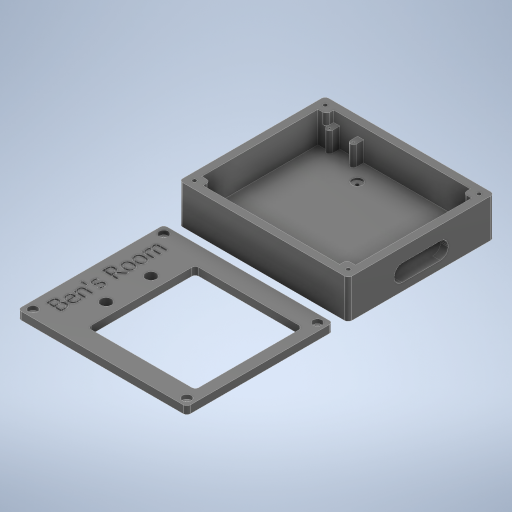
# Autodesk Inventor part: Front Circuit Box
Saved by Autodesk Inventor 2024 (Build 280153000, 153)
## iProperties
Created: 2024-01-30
Part Number: Front Circuit Box
Material: ABS Plastic
Document SubType Name: Modeling
Designer: himmelb
Density: 1.06 g/cm^3
Appearance: Smooth - Black
Author: himmelb
Autodesk Inventor part; units mm, degrees
ref_plane "YZ Plane" through (0, 0, 0) normal (1, 0, 0) x (0, 1, 0)
ref_plane "XZ Plane" through (0, 0, 0) normal (0, 1, 0) x (-1, 0, 0)
ref_plane "XY Plane" through (0, 0, 0) normal (0, 0, 1) x (1, 0, 0)
sketch "Sketch1" plane through (0, 0, 0) normal (0, 1, 0) x (-1, 0, 0)
  line L0 (0, 0) -> (110, 0)
  line L1 (110, 0) -> (110, -95)
  line L2 (110, -95) -> (0, -95)
  line L3 (0, -95) -> (0, 0)
  dimension "d0" = 110
  dimension "d1" = 95
  constraints: 8 end point, 2 parallel, 1 horizontal, 1 perpendicular
  measures "d0" distance of L1.end L2.end
  measures "d1" distance of L0.end L1.end
extrude "Extrusion1" add sketch "Sketch1" along normal blind 25
shell "Shell1" thickness 5 removed faces 1 at (-36.6667, 25, -31.6667)
sketch "Sketch2" plane through (-105, 5, -90) normal (0, 1, 0) x (1, 0, 0)
  circle A0 centre (92, -72.1) radius 3.5
  circle A1 centre (92, -12.9) radius 3.5
  circle A2 centre (33.73, -72.0689) radius 3.5
  circle A3 centre (33.73, -12.9) radius 3.5
  line L0 (100, -85) -> (0, -85) projected
  line L1 (0, 0) -> (100, 0) projected
  line L2 (100, 0) -> (100, -85) projected
  point P0 (105, -90)
  dimension "d8" = 58.27
  dimension "d9" = 12.9
  dimension "d10" = 12.9
  dimension "d11" = 8
  dimension "d13" = 8
  dimension "d15" = 7
  dimension "d16" = 7
  dimension "d17" = 7
  dimension "d18" = 7
  constraints: 4 centre point
  measures "d8" distance of A0.centre A2.centre
  measures "d9" distance from line of A0.centre L0
  measures "d10" distance from line of L1 A1.centre
  measures "d11" distance from line of L2 A0.centre
  measures "d13" distance from line of L2 A1.centre
  measures "d15" diameter of A2
  measures "d16" diameter of A3
  measures "d17" diameter of A0
  measures "d18" diameter of A1
extrude "Extrusion2" cut sketch "Sketch2" against normal blind 1.5
sketch "Sketch3" plane through (0, 0, 0) normal (0, -1, 0) x (1, 0, 0)
  circle A0 centre (-13, -17.9) radius 3.5 projected
  circle A1 centre (-13, -17.9) radius 3.5
  circle A2 centre (-13, -77.1) radius 3.5 projected
  circle A3 centre (-13, -77.1) radius 3.5
  circle A4 centre (-71.27, -77.1) radius 3.5 projected
  circle A5 centre (-71.27, -77.1) radius 3.5
  circle A6 centre (-71.27, -17.9311) radius 3.5 projected
  circle A7 centre (-71.27, -17.9311) radius 3.5
  point P0 (0, 0)
  constraints: 4 centre point, 4 coincident
extrude "Extrusion3" cut sketch "Sketch3" against normal blind 1.5
sketch "Sketch4" plane through (-71.27, 3.5, -77.1) normal (0, 1, 0) x (1, 0, 0)
  circle A0 centre (0, 0) radius 3.5 projected
  circle A1 centre (0, 0) radius 1.25
  circle A2 centre (0, -59.1689) radius 3.5 projected
  circle A3 centre (0, -59.1689) radius 1.25
  circle A4 centre (58.27, -59.2) radius 3.5 projected
  circle A5 centre (58.27, -59.2) radius 1.25
  circle A6 centre (58.27, 0) radius 3.5 projected
  circle A7 centre (58.27, 0) radius 1.25
  point P0 (71.27, -77.1)
  dimension "d24" = 2.5
  dimension "d25" = 2.5
  dimension "d26" = 2.5
  dimension "d27" = 2.5
  constraints: 4 centre point, 4 coincident
  measures "d24" diameter of A1
  measures "d25" diameter of A7
  measures "d26" diameter of A5
  measures "d27" diameter of A3
extrude "Extrusion4" cut sketch "Sketch4" against normal blind 2 contours A1 | A3 | A5 | A7
sketch "Sketch5" plane through (0, 0, 0) normal (1, 0, 0) x (0, 0, -1)
  line L0 (95, 0) -> (0, 0) projected
  line L1 (65, 5) -> (65, 16.0603)
  line L2 (65, 16.0603) -> (30, 16.0603)
  line L3 (30, 16.0603) -> (30, 5)
  line L4 (0, 0) -> (0, 25) projected
  line L5 (30, 5) -> (65, 5)
  dimension "d33" = 35
  dimension "d34" = 30
  dimension "d35" = 5
  constraints: 8 end point, 1 parallel, 1 perpendicular
  measures "d33" distance between parallel lines of L1 L3
  measures "d34" distance between parallel lines of L4 L3
  measures "d35" distance between parallel lines of L5 L0
extrude "Extrusion5" cut sketch "Sketch5" against normal blind 5
sketch "Sketch6" plane through (-105, 5, -90) normal (0, 1, 0) x (1, 0, 0)
  circle A0 centre (33.73, -72.0689) radius 3.5 projected
  line L0 (0, 0) -> (0, -85) projected
  circle A1 centre (33.73, -12.9) radius 3.5 projected
  line L1 (100, -85) -> (0, -85) projected
  line L2 (0, 0) -> (100, 0) projected
  arc A2 (9.5575, -80.25) -> (5.5575, -80.25) centre (7.5575, -80.25) ccw
  arc A3 (25.0575, -80.25) -> (21.0575, -80.25) centre (23.0575, -80.25) ccw
  arc A4 (21.0575, -4.75) -> (25.0575, -4.75) centre (23.0575, -4.75) ccw
  arc A5 (5.5575, -4.75) -> (9.5575, -4.75) centre (7.5575, -4.75) ccw
  line L3 (25.0575, -80.25) -> (25.0575, -85)
  line L4 (25.0575, -85) -> (5.5575, -85)
  line L5 (5.5575, -85) -> (5.5575, -80.25)
  line L6 (25.0575, -4.75) -> (25.0575, 0)
  line L7 (25.0575, 0) -> (5.5575, 0)
  line L8 (5.5575, 0) -> (5.5575, -4.75)
  line L9 (9.5575, -80.25) -> (9.5575, -85)
  line L10 (21.0575, -80.25) -> (21.0575, -85)
  line L11 (21.0575, -4.75) -> (21.0575, 0)
  line L12 (9.5575, -4.75) -> (9.5575, 0)
  line L13 (5.5575, -80.25) -> (9.5575, -80.25)
  line L14 (21.0575, -80.25) -> (25.0575, -80.25)
  point P0 (105, -90)
  point P1 (21.0575, -85)
  point P2 (5.5575, -85)
  point P3 (9.5575, -85)
  point P4 (21.0575, 0)
  dimension "d39" = 4.75
  dimension "d40" = 4.75
  dimension "d41" = 4.75
  dimension "d42" = 4.75
  dimension "d43" = 15.5
  dimension "d44" = 15.5
  dimension "d45" = 4
  dimension "d46" = 4
  dimension "d47" = 4
  dimension "d48" = 4
  constraints: 24 end point, 9 point on line, 8 point on circle, 4 centre point, 4 coincident, 4 parallel, 3 perpendicular, 2 horizontal, 2 tangent
  measures "d39" distance from line of L1 point (7.558, -80.25)
  measures "d40" distance from line of L2 point (7.558, -4.75)
  measures "d41" distance from line of L2 point (23.058, -4.75)
  measures "d42" distance from line of L1 point (23.058, -80.25)
  measures "d43" distance of point (23.058, -80.25) point (7.558, -80.25)
  measures "d44" distance of point (23.058, -4.75) point (7.558, -4.75)
  measures "d45" diameter of A5
  measures "d46" diameter of A4
  measures "d47" diameter of A3
  measures "d48" diameter of A2
extrude "Extrusion6" add sketch "Sketch6" along normal blind 13 contours L1 L10 L14 L3 | L14 A3 | L1 L5 L13 L9 | L13 A2 | L2 L12 A5 L8 | L2 L6 A4 L11
sketch "Sketch7" plane through (-97.4425, 18, -9.75) normal (0, 1, 0) x (-1, 0, 0)
  circle A0 centre (0, 0) radius 0.64
  arc A1 (-17.5, 0) -> (-13.5, 0) centre (-15.5, 0) ccw projected
  circle A2 centre (-15.5, 0) radius 0.64
  arc A3 (2, -75.5) -> (-2, -75.5) centre (0, -75.5) ccw projected
  circle A4 centre (0, -75.5) radius 0.64
  arc A5 (-13.5, -75.5) -> (-17.5, -75.5) centre (-15.5, -75.5) ccw projected
  circle A6 centre (-15.5, -75.5) radius 0.64
  point P0 (-97.4425, 9.75)
  point P1 (15.5, 0)
  point P2 (15.5, 75.5)
  point P3 (0, 75.5)
  dimension "d51" = 1.28
  dimension "d52" = 1.28
  dimension "d53" = 1.28
  dimension "d54" = 1.28
  constraints: 4 centre point, 4 coincident
  measures "d51" diameter of A6
  measures "d52" diameter of A4
  measures "d53" diameter of A2
  measures "d54" diameter of A0
extrude "Extrusion7" cut sketch "Sketch7" against normal blind 5.4
sketch "Sketch8" plane through (0, 25, 0) normal (0, 1, 0) x (1, 0, 0)
  line L0 (-105, 5) -> (-105, 90) projected
  arc A0 (-95.4425, 9.75) -> (-99.4425, 9.75) centre (-97.4425, 9.75) ccw projected
  line L1 (-105, 5) -> (-99.4425, 5)
  line L2 (-99.4425, 5) -> (-99.4425, 9.75)
  line L3 (-99.4425, 9.75) -> (-105, 9.75)
  line L4 (-105, 9.75) -> (-105, 5)
  arc A1 (-99.4425, 85.25) -> (-95.4425, 85.25) centre (-97.4425, 85.25) ccw projected
  line L5 (-105, 90) -> (-99.4425, 90)
  line L6 (-99.4425, 90) -> (-99.4425, 85.25)
  line L7 (-99.4425, 85.25) -> (-105, 85.25)
  line L8 (-105, 85.25) -> (-105, 90)
  line L9 (-105, 5) -> (-5, 5) projected
  line L10 (-55, 5) -> (-55, 90)
  line L11 (-5, 90) -> (-105, 90) projected
  line L12 (-5, 5) -> (-10.5575, 5)
  line L13 (-10.5575, 5) -> (-10.5575, 9.75)
  line L14 (-10.5575, 9.75) -> (-5, 9.75)
  line L15 (-5, 9.75) -> (-5, 5)
  line L16 (-5, 90) -> (-10.5575, 90)
  line L17 (-10.5575, 90) -> (-10.5575, 85.25)
  line L18 (-10.5575, 85.25) -> (-5, 85.25)
  line L19 (-5, 85.25) -> (-5, 90)
  line L20 (-5, 5) -> (-5, 9.75)
  line L21 (-5, 85.25) -> (-5, 90)
  point P0 (0, 0)
  constraints: 38 end point, 6 symmetric about line, 4 parallel, 2 horizontal, 2 midpoint, 2 perpendicular, 2 point on circle
extrude "Extrusion8" add sketch "Sketch8" against normal blind 20 contours L0 L3 L2 L1 | L0 L5 L6 L7 | L13 L14 L15 L9 | L19 L18 L17 L11
fillet "Fillet1" radius 5.08 4 edges at (-2.5, 16.0603, -65) (-2.5, 16.0603, -30) (-2.5, 5, -30) (-2.5, 5, -65)
sketch "Sketch9" plane through (0, 25, 0) normal (0, 1, 0) x (1, 0, 0)
  circle A0 centre (-105, 90) radius 1.335
  circle A1 centre (-5, 90) radius 1.335
  circle A2 centre (-5, 5) radius 1.335
  circle A3 centre (-105, 5) radius 1.335
  line L0 (-99.4425, 85.25) -> (-99.4425, 90) projected
  line L1 (-105, 85.25) -> (-99.4425, 85.25) projected
  point P0 (0, 0)
  point P1 (-102.2212, 85.25)
  dimension "d65" = 2.67
  dimension "d66" = 2.67
  dimension "d67" = 2.67
  dimension "d68" = 2.67
  constraints: 4 centre point, 1 midpoint
  measures "d65" diameter of A0
  measures "d66" diameter of A1
  measures "d67" diameter of A2
  measures "d68" diameter of A3
extrude "Extrusion9" cut sketch "Sketch9" against normal blind 20
sketch "Sketch10" plane through (0, 0, 0) normal (0, -1, 0) x (1, 0, 0)
  line L0 (0, 105) -> (-110, 105)
  line L1 (-110, 105) -> (-110, 10)
  line L2 (-110, 10) -> (0, 10)
  line L3 (0, 10) -> (0, 105)
  line L4 (0, 0) -> (0, -95) projected
  line L5 (-110, 0) -> (0, 0) projected
  dimension "d71" = 95
  dimension "d72" = 110
  dimension "d73" = 0
  dimension "d74" = 10
  constraints: 8 end point, 2 parallel, 1 horizontal, 1 perpendicular
  measures "d71" distance between parallel lines of L2 L0
  measures "d72" distance of L1.end L2.end
  measures "d73" distance between parallel lines of L3 L4
  measures "d74" distance between parallel lines of L5 L2
extrude "Extrusion10" add sketch "Sketch10" against normal blind 5
sketch "Sketch11" plane through (0, 5, 0) normal (0, 1, 0) x (1, 0, 0)
  circle A0 centre (-105, -15) radius 1.335
  circle A1 centre (-5, -15) radius 1.335
  circle A2 centre (-5, -100) radius 1.335
  circle A3 centre (-105, -100) radius 1.335
  line L0 (0, -10) -> (-110, -10) projected
  line L1 (0, -105) -> (0, -10) projected
  line L2 (-110, -105) -> (0, -105) projected
  line L3 (-110, -10) -> (-110, -105) projected
  circle A4 centre (-105, -15) radius 3
  circle A5 centre (-5, -15) radius 3
  circle A6 centre (-5, -100) radius 3
  circle A7 centre (-105, -100) radius 3
  point P0 (0, 0)
  dimension "d77" = 5
  dimension "d78" = 5
  dimension "d79" = 5
  dimension "d80" = 5
  dimension "d81" = 5
  dimension "d82" = 5
  dimension "d83" = 5
  dimension "d84" = 5
  dimension "d85" = 2.67
  dimension "d86" = 2.67
  dimension "d87" = 2.67
  dimension "d88" = 2.67
  dimension "d89" = 6
  dimension "d90" = 6
  dimension "d91" = 6
  dimension "d92" = 6
  constraints: 8 centre point, 4 coincident
  measures "d77" distance from line of L0 A1.centre
  measures "d78" distance from line of L1 A1.centre
  measures "d79" distance from line of L2 A2.centre
  measures "d80" distance from line of L1 A2.centre
  measures "d81" distance from line of L2 A3.centre
  measures "d82" distance from line of L3 A3.centre
  measures "d83" distance from line of L3 A0.centre
  measures "d84" distance from line of L0 A0.centre
  measures "d85" diameter of A3
  measures "d86" diameter of A0
  measures "d87" diameter of A1
  measures "d88" diameter of A2
  measures "d89" diameter of A4
  measures "d90" diameter of A5
  measures "d91" diameter of A6
  measures "d92" diameter of A7
extrude "Extrusion11" cut sketch "Sketch11" against normal blind 2.7 contours A0 | A1 | A2 | A3 | A4 | A5 | A6 | A7
sketch "Sketch12" plane through (0, 5, 0) normal (0, 1, 0) x (1, 0, 0)
  circle A0 centre (-105, -100) radius 3 projected
  circle A1 centre (-105, -100) radius 1.335
  circle A2 centre (-105, -15) radius 3 projected
  circle A3 centre (-105, -15) radius 1.335
  circle A4 centre (-5, -15) radius 3 projected
  circle A5 centre (-5, -15) radius 1.335
  circle A6 centre (-5, -100) radius 3 projected
  circle A7 centre (-5, -100) radius 1.335
  line L0 (-110, -10) -> (-110, -105) projected
  point P0 (0, 0)
  dimension "d95" = 2.67
  dimension "d96" = 2.67
  dimension "d97" = 2.67
  dimension "d98" = 2.67
  constraints: 4 centre point, 4 coincident
  measures "d95" diameter of A1
  measures "d96" diameter of A3
  measures "d97" diameter of A5
  measures "d98" diameter of A7
extrude "Extrusion12" cut sketch "Sketch12" against normal blind 5 contours A1 | A3 | A5 | A7
sketch "Sketch13" plane through (0, 5, 0) normal (0, 1, 0) x (1, 0, 0)
  line L0 (-77, -22.5) -> (-7, -22.5)
  line L1 (-7, -22.5) -> (-7, -92.5)
  line L2 (-7, -92.5) -> (-77, -92.5)
  line L3 (-77, -92.5) -> (-77, -22.5)
  line L4 (0, -10) -> (-110, -10) projected
  line L5 (0, -105) -> (0, -10) projected
  circle A0 centre (-13, 17.9) radius 3.5 projected
  circle A1 centre (-71.27, 17.9311) radius 3.5 projected
  circle A2 centre (-85.4425, -42.89) radius 3.5
  circle A3 centre (-85.4425, -72.11) radius 3.5
  line L6 (-110, -105) -> (0, -105) projected
  circle A4 centre (-81.9425, 9.75) radius 0.64 projected
  circle A5 centre (-97.4425, 9.75) radius 0.64 projected
  point P0 (0, 0)
  dimension "d101" = 70
  dimension "d102" = 70
  dimension "d103" = 12.5
  dimension "d104" = 7
  dimension "d105" = 7
  dimension "d106" = 7
  dimension "d107" = 32.89
  dimension "d108" = 32.89
  dimension "d110" = 3.5
  dimension "d111" = 3.5
  constraints: 8 end point, 3 coincident, 2 centre point, 2 parallel, 1 horizontal, 1 perpendicular
  measures "d101" distance between parallel lines of L2 L0
  measures "d102" distance of L0.start L0.end
  measures "d103" distance between parallel lines of L4 L0
  measures "d104" distance between parallel lines of L5 L1
  measures "d105" diameter of A2
  measures "d106" diameter of A3
  measures "d107" distance from line of L4 A2.centre
  measures "d108" distance from line of L6 A3.centre
  measures "d110" horizontal distance of A2.centre point (-81.942, 9.75)
  measures "d111" horizontal distance of point (-81.942, 9.75) A3.centre
extrude "Extrusion13" cut sketch "Sketch13" against normal blind 5 contours L0 L1 L2 L3 | A2 | A3
fillet "Fillet3" radius 2.25 16 edges at (0, 2.5, 105) (0, 2.5, 10) (-110, 2.5, 105) (-77, 2.5, 22.5) (-7, 2.5, 22.5) (-7, 2.5, 92.5) (-77, 2.5, 92.5) (-110, 2.5, 10) (-110, 12.5, -95) (0, 12.5, -95) (-110, 12.5, 0) (0, 12.5, 0) (-99.4425, 21.5, -9.75) (-99.4425, 21.5, -85.25) (-10.5575, 15, -85.25) (-10.5575, 15, -9.75)
sketch "Sketch14" plane through (0, 5, 0) normal (0, 1, 0) x (1, 0, 0)
  line L0 (-105, -95) -> (-105, -20) construction
  line L1 (-105, -20) -> (-90.6726, -20) construction
  line L2 (-90.6726, -20) -> (-90.6726, -95) construction
  line L3 (-90.6726, -95) -> (-105, -95) construction
  line L4 (-110, -12.25) -> (-110, -102.75) projected
  line L5 (-107.75, -105) -> (-2.25, -105) projected
  line L6 (-2.25, -10) -> (-107.75, -10) projected
  spline S0 degree 2 poles (-97.62, -85.398) (-96.8739, -85.398) (-95.7304, -85.9657) (-95.3573, -86.4361) knots 0 0 0 1 2 2 2
  spline S1 degree 2 poles (-95.3573, -86.4361) (-94.9194, -87.0038) (-94.5464, -88.2932) (-94.5464, -89.3151) knots 0 0 0 1 2 2 2
  line L7 (-94.5464, -89.3151) -> (-94.5464, -92.186)
  line L8 (-94.5464, -92.186) -> (-104.554, -92.186)
  line L9 (-104.554, -92.186) -> (-104.554, -89.534)
  spline S2 degree 2 poles (-104.554, -89.534) (-104.554, -88.4635) (-104.4161, -87.393) (-104.1485, -86.9064) knots 0 0 0 1 2 2 2
  spline S3 degree 2 poles (-104.1485, -86.9064) (-103.8646, -86.3631) (-102.932, -85.8684) (-102.2994, -85.8684) knots 0 0 0 1 2 2 2
  spline S4 degree 2 poles (-102.2994, -85.8684) (-101.5938, -85.8684) (-100.4747, -86.6145) (-100.1584, -87.2714) knots 0 0 0 1 2 2 2
  line L10 (-100.1584, -87.2714) -> (-100.1097, -87.2714)
  spline S5 degree 2 poles (-100.1097, -87.2714) (-99.8664, -86.3793) (-98.577, -85.398) (-97.62, -85.398) knots 0 0 0 1 2 2 2
  spline S6 degree 2 poles (-97.5632, -86.7848) (-98.1309, -86.7848) (-98.8608, -87.1092) (-99.1203, -87.5958) knots 0 0 0 1 2 2 2
  spline S7 degree 2 poles (-99.1203, -87.5958) (-99.2825, -87.9121) (-99.3798, -88.6582) (-99.3798, -89.3475) knots 0 0 0 1 2 2 2
  line L11 (-99.3798, -89.3475) -> (-99.3798, -90.856)
  line L12 (-99.3798, -90.856) -> (-95.6817, -90.856)
  line L13 (-95.6817, -90.856) -> (-95.6817, -89.7773)
  spline S8 degree 2 poles (-95.6817, -89.7773) (-95.6817, -88.9015) (-95.8439, -87.8959) (-96.1035, -87.5066) knots 0 0 0 1 2 2 2
  spline S9 degree 2 poles (-96.1035, -87.5066) (-96.3711, -87.1335) (-97.0361, -86.7848) (-97.5632, -86.7848) knots 0 0 0 1 2 2 2
  spline S10 degree 2 poles (-102.1129, -87.2552) (-102.4697, -87.2552) (-103.005, -87.4985) (-103.1591, -87.7661) knots 0 0 0 1 2 2 2
  spline S11 degree 2 poles (-103.1591, -87.7661) (-103.3375, -88.0905) (-103.4186, -88.8771) (-103.4186, -89.5827) knots 0 0 0 1 2 2 2
  line L14 (-103.4186, -89.5827) -> (-103.4186, -90.856)
  line L15 (-103.4186, -90.856) -> (-100.4909, -90.856)
  line L16 (-100.4909, -90.856) -> (-100.4909, -89.3475)
  spline S12 degree 2 poles (-100.4909, -89.3475) (-100.4909, -88.7231) (-100.6207, -88.131) (-100.8234, -87.8148) knots 0 0 0 1 2 2 2
  spline S13 degree 2 poles (-100.8234, -87.8148) (-101.018, -87.5066) (-101.6425, -87.2552) (-102.1129, -87.2552) knots 0 0 0 1 2 2 2
  spline S14 degree 2 poles (-94.376, -80.9132) (-94.376, -82.7136) (-96.3954, -84.6924) (-98.2607, -84.6924) knots 0 0 0 1 2 2 2
  spline S15 degree 2 poles (-98.2607, -84.6924) (-100.0935, -84.6924) (-102.267, -82.7704) (-102.267, -81.2214) knots 0 0 0 1 2 2 2
  spline S16 degree 2 poles (-102.267, -81.2214) (-102.267, -80.524) (-101.8615, -79.4454) (-101.4317, -79.048) knots 0 0 0 1 2 2 2
  spline S17 degree 2 poles (-101.4317, -79.048) (-101.0018, -78.6425) (-99.761, -78.2126) (-98.8608, -78.2126) knots 0 0 0 1 2 2 2
  line L17 (-98.8608, -78.2126) -> (-98.1715, -78.2126)
  line L18 (-98.1715, -78.2126) -> (-98.1715, -83.4111)
  spline S18 degree 2 poles (-98.1715, -83.4111) (-96.8658, -83.4111) (-95.479, -82.0973) (-95.479, -80.9295) knots 0 0 0 1 2 2 2
  spline S19 degree 2 poles (-95.479, -80.9295) (-95.479, -80.5159) (-95.6655, -79.713) (-95.8115, -79.3886) knots 0 0 0 1 2 2 2
  spline S20 degree 2 poles (-95.8115, -79.3886) (-95.9737, -79.048) (-96.2575, -78.5776) (-96.3873, -78.4235) knots 0 0 0 1 2 2 2
  line L19 (-96.3873, -78.4235) -> (-96.3873, -78.3505)
  line L20 (-96.3873, -78.3505) -> (-95.0086, -78.3505)
  spline S21 degree 2 poles (-95.0086, -78.3505) (-94.9194, -78.5695) (-94.6599, -79.2345) (-94.5869, -79.494) knots 0 0 0 1 2 2 2
  spline S22 degree 2 poles (-94.5869, -79.494) (-94.4815, -79.859) (-94.376, -80.4591) (-94.376, -80.9132) knots 0 0 0 1 2 2 2
  spline S23 degree 2 poles (-99.1366, -79.4454) (-99.6475, -79.4616) (-100.3936, -79.6724) (-100.645, -79.8752) knots 0 0 0 1 2 2 2
  spline S24 degree 2 poles (-100.645, -79.8752) (-100.9288, -80.0941) (-101.2289, -80.7835) (-101.2289, -81.2944) knots 0 0 0 1 2 2 2
  spline S25 degree 2 poles (-101.2289, -81.2944) (-101.2289, -81.7972) (-100.9288, -82.5028) (-100.6369, -82.7947) knots 0 0 0 1 2 2 2
  spline S26 degree 2 poles (-100.6369, -82.7947) (-100.3368, -83.0786) (-99.615, -83.3705) (-99.1366, -83.4111) knots 0 0 0 1 2 2 2
  line L21 (-99.1366, -83.4111) -> (-99.1366, -79.4454)
  line L22 (-94.5464, -71.0354) -> (-94.5464, -72.3005)
  line L23 (-94.5464, -72.3005) -> (-98.8284, -72.3005)
  spline S27 degree 2 poles (-98.8284, -72.3005) (-99.3474, -72.3005) (-100.2395, -72.3979) (-100.5071, -72.5438) knots 0 0 0 1 2 2 2
  spline S28 degree 2 poles (-100.5071, -72.5438) (-100.791, -72.6979) (-101.0667, -73.2494) (-101.0667, -73.7198) knots 0 0 0 1 2 2 2
  spline S29 degree 2 poles (-101.0667, -73.7198) (-101.0667, -74.1901) (-100.5639, -75.1877) (-100.1584, -75.6661) knots 0 0 0 1 2 2 2
  line L24 (-100.1584, -75.6661) -> (-94.5464, -75.6661)
  line L25 (-94.5464, -75.6661) -> (-94.5464, -76.9313)
  line L26 (-94.5464, -76.9313) -> (-102.0561, -76.9313)
  line L27 (-102.0561, -76.9313) -> (-102.0561, -75.6661)
  line L28 (-102.0561, -75.6661) -> (-101.2208, -75.6661)
  spline S30 degree 2 poles (-101.2208, -75.6661) (-101.7317, -75.0985) (-102.267, -74.0036) (-102.267, -73.3873) knots 0 0 0 1 2 2 2
  spline S31 degree 2 poles (-102.267, -73.3873) (-102.267, -72.2843) (-100.8072, -71.0354) (-99.4204, -71.0354) knots 0 0 0 1 2 2 2
  line L29 (-99.4204, -71.0354) -> (-94.5464, -71.0354)
  line L30 (-105, -67.978) -> (-101.1073, -68.2699)
  line L31 (-101.1073, -68.2699) -> (-101.1073, -69.1782)
  line L32 (-101.1073, -69.1782) -> (-105, -69.4702)
  line L33 (-105, -69.4702) -> (-105, -67.978)
  spline S32 degree 2 poles (-94.3679, -64.3285) (-94.3679, -65.0827) (-94.7734, -66.3884) (-95.0005, -66.8183) knots 0 0 0 1 2 2 2
  line L34 (-95.0005, -66.8183) -> (-96.4197, -66.8183)
  line L35 (-96.4197, -66.8183) -> (-96.4197, -66.7534)
  spline S33 degree 2 poles (-96.4197, -66.7534) (-96.29, -66.5912) (-95.9818, -66.1532) (-95.8115, -65.7883) knots 0 0 0 1 2 2 2
  spline S34 degree 2 poles (-95.8115, -65.7883) (-95.6574, -65.472) (-95.4303, -64.6935) (-95.4303, -64.2799) knots 0 0 0 1 2 2 2
  spline S35 degree 2 poles (-95.4303, -64.2799) (-95.4303, -63.9798) (-95.5682, -63.2905) (-95.6817, -63.1283) knots 0 0 0 1 2 2 2
  spline S36 degree 2 poles (-95.6817, -63.1283) (-95.8358, -62.8931) (-96.1846, -62.6822) (-96.5414, -62.6822) knots 0 0 0 1 2 2 2
  spline S37 degree 2 poles (-96.5414, -62.6822) (-96.9874, -62.6822) (-97.4497, -63.1688) (-97.6038, -63.7933) knots 0 0 0 1 2 2 2
  spline S38 degree 2 poles (-97.6038, -63.7933) (-97.6606, -64.0366) (-97.8228, -64.8151) (-97.912, -65.1476) knots 0 0 0 1 2 2 2
  spline S39 degree 2 poles (-97.912, -65.1476) (-98.1634, -66.0073) (-99.2014, -66.7858) (-99.9394, -66.7858) knots 0 0 0 1 2 2 2
  spline S40 degree 2 poles (-99.9394, -66.7858) (-100.9613, -66.7858) (-102.2345, -65.2531) (-102.2345, -63.9879) knots 0 0 0 1 2 2 2
  spline S41 degree 2 poles (-102.2345, -63.9879) (-102.2345, -63.3634) (-101.9264, -62.0983) (-101.6912, -61.6685) knots 0 0 0 1 2 2 2
  line L36 (-101.6912, -61.6685) -> (-100.3368, -61.6685)
  line L37 (-100.3368, -61.6685) -> (-100.3368, -61.7334)
  spline S42 degree 2 poles (-100.3368, -61.7334) (-100.7261, -62.22) (-101.1721, -63.404) (-101.1721, -64.0122) knots 0 0 0 1 2 2 2
  spline S43 degree 2 poles (-101.1721, -64.0122) (-101.1721, -64.6367) (-100.645, -65.4963) (-100.1178, -65.4963) knots 0 0 0 1 2 2 2
  spline S44 degree 2 poles (-100.1178, -65.4963) (-99.6394, -65.4963) (-99.1771, -64.9854) (-99.0311, -64.4177) knots 0 0 0 1 2 2 2
  spline S45 degree 2 poles (-99.0311, -64.4177) (-98.9581, -64.142) (-98.8122, -63.4445) (-98.7229, -63.0634) knots 0 0 0 1 2 2 2
  spline S46 degree 2 poles (-98.7229, -63.0634) (-98.5121, -62.2362) (-97.547, -61.3927) (-96.7117, -61.3927) knots 0 0 0 1 2 2 2
  spline S47 degree 2 poles (-96.7117, -61.3927) (-96.2251, -61.3927) (-95.3655, -61.7739) (-95.0492, -62.147) knots 0 0 0 1 2 2 2
  spline S48 degree 2 poles (-95.0492, -62.147) (-94.7167, -62.5443) (-94.3679, -63.5581) (-94.3679, -64.3285) knots 0 0 0 1 2 2 2
  line L38 (-94.5464, -48.0763) -> (-94.5464, -49.8037)
  line L39 (-94.5464, -49.8037) -> (-98.5283, -52.9666)
  line L40 (-98.5283, -52.9666) -> (-98.5283, -54.4912)
  line L41 (-98.5283, -54.4912) -> (-94.5464, -54.4912)
  line L42 (-94.5464, -54.4912) -> (-94.5464, -55.8213)
  line L43 (-94.5464, -55.8213) -> (-104.554, -55.8213)
  line L44 (-104.554, -55.8213) -> (-104.554, -53.2423)
  spline S49 degree 2 poles (-104.554, -53.2423) (-104.554, -52.3827) (-104.3674, -51.2229) (-104.0268, -50.6958) knots 0 0 0 1 2 2 2
  spline S50 degree 2 poles (-104.0268, -50.6958) (-103.6862, -50.1687) (-102.6238, -49.5604) (-101.8371, -49.5604) knots 0 0 0 1 2 2 2
  spline S51 degree 2 poles (-101.8371, -49.5604) (-100.7423, -49.5604) (-99.2582, -50.6796) (-98.9014, -51.6366) knots 0 0 0 1 2 2 2
  line L45 (-98.9014, -51.6366) -> (-94.5464, -48.0763)
  spline S52 degree 2 poles (-101.7317, -50.9472) (-102.1697, -50.9472) (-102.8428, -51.2554) (-103.0617, -51.5798) knots 0 0 0 1 2 2 2
  spline S53 degree 2 poles (-103.0617, -51.5798) (-103.2483, -51.8636) (-103.4024, -52.6178) (-103.4024, -53.1693) knots 0 0 0 1 2 2 2
  line L46 (-103.4024, -53.1693) -> (-103.4024, -54.4912)
  line L47 (-103.4024, -54.4912) -> (-99.6394, -54.4912)
  line L48 (-99.6394, -54.4912) -> (-99.6394, -53.3234)
  spline S54 degree 2 poles (-99.6394, -53.3234) (-99.6394, -52.7476) (-99.8421, -51.8312) (-100.1584, -51.5149) knots 0 0 0 1 2 2 2
  spline S55 degree 2 poles (-100.1584, -51.5149) (-100.4341, -51.2229) (-101.2127, -50.9472) (-101.7317, -50.9472) knots 0 0 0 1 2 2 2
  spline S56 degree 2 poles (-98.3012, -41.2072) (-96.4035, -41.2072) (-94.3355, -43.032) (-94.3355, -44.5566) knots 0 0 0 1 2 2 2
  spline S57 degree 2 poles (-94.3355, -44.5566) (-94.3355, -46.1218) (-96.4684, -47.9141) (-98.3012, -47.9141) knots 0 0 0 1 2 2 2
  spline S58 degree 2 poles (-98.3012, -47.9141) (-100.1827, -47.9141) (-102.267, -46.0651) (-102.267, -44.5566) knots 0 0 0 1 2 2 2
  spline S59 degree 2 poles (-102.267, -44.5566) (-102.267, -43.032) (-100.1908, -41.2072) (-98.3012, -41.2072) knots 0 0 0 1 2 2 2
  spline S60 degree 2 poles (-98.3012, -42.5129) (-99.761, -42.5129) (-101.1802, -43.5753) (-101.1802, -44.5566) knots 0 0 0 1 2 2 2
  spline S61 degree 2 poles (-101.1802, -44.5566) (-101.1802, -45.5379) (-99.761, -46.6084) (-98.3012, -46.6084) knots 0 0 0 1 2 2 2
  spline S62 degree 2 poles (-98.3012, -46.6084) (-96.882, -46.6084) (-95.4222, -45.5379) (-95.4222, -44.5566) knots 0 0 0 1 2 2 2
  spline S63 degree 2 poles (-95.4222, -44.5566) (-95.4222, -43.5834) (-96.8577, -42.5129) (-98.3012, -42.5129) knots 0 0 0 1 2 2 2
  spline S64 degree 2 poles (-98.3012, -33.738) (-96.4035, -33.738) (-94.3355, -35.5628) (-94.3355, -37.0874) knots 0 0 0 1 2 2 2
  spline S65 degree 2 poles (-94.3355, -37.0874) (-94.3355, -38.6526) (-96.4684, -40.4449) (-98.3012, -40.4449) knots 0 0 0 1 2 2 2
  spline S66 degree 2 poles (-98.3012, -40.4449) (-100.1827, -40.4449) (-102.267, -38.5959) (-102.267, -37.0874) knots 0 0 0 1 2 2 2
  spline S67 degree 2 poles (-102.267, -37.0874) (-102.267, -35.5628) (-100.1908, -33.738) (-98.3012, -33.738) knots 0 0 0 1 2 2 2
  spline S68 degree 2 poles (-98.3012, -35.0437) (-99.761, -35.0437) (-101.1802, -36.1061) (-101.1802, -37.0874) knots 0 0 0 1 2 2 2
  spline S69 degree 2 poles (-101.1802, -37.0874) (-101.1802, -38.0687) (-99.761, -39.1392) (-98.3012, -39.1392) knots 0 0 0 1 2 2 2
  spline S70 degree 2 poles (-98.3012, -39.1392) (-96.882, -39.1392) (-95.4222, -38.0687) (-95.4222, -37.0874) knots 0 0 0 1 2 2 2
  spline S71 degree 2 poles (-95.4222, -37.0874) (-95.4222, -36.1142) (-96.8577, -35.0437) (-98.3012, -35.0437) knots 0 0 0 1 2 2 2
  line L49 (-94.5464, -23.9251) -> (-98.8933, -23.9251)
  spline S72 degree 2 poles (-98.8933, -23.9251) (-99.4123, -23.9251) (-100.2963, -24.0062) (-100.5396, -24.1359) knots 0 0 0 1 2 2 2
  spline S73 degree 2 poles (-100.5396, -24.1359) (-100.8072, -24.2657) (-101.0667, -24.7604) (-101.0667, -25.1902) knots 0 0 0 1 2 2 2
  spline S74 degree 2 poles (-101.0667, -25.1902) (-101.0667, -25.5795) (-100.5882, -26.4716) (-100.1341, -26.9419) knots 0 0 0 1 2 2 2
  spline S75 degree 2 poles (-100.1341, -26.9419) (-100.0205, -26.9338) (-99.7042, -26.9176) (-99.4934, -26.9176) knots 0 0 0 1 2 2 2
  line L50 (-99.4934, -26.9176) -> (-94.5464, -26.9176)
  line L51 (-94.5464, -26.9176) -> (-94.5464, -28.1828)
  line L52 (-94.5464, -28.1828) -> (-98.8933, -28.1828)
  spline S76 degree 2 poles (-98.8933, -28.1828) (-99.4123, -28.1828) (-100.2963, -28.2639) (-100.5396, -28.3936) knots 0 0 0 1 2 2 2
  spline S77 degree 2 poles (-100.5396, -28.3936) (-100.8072, -28.5234) (-101.0667, -29.0181) (-101.0667, -29.4479) knots 0 0 0 1 2 2 2
  spline S78 degree 2 poles (-101.0667, -29.4479) (-101.0667, -29.8534) (-100.5558, -30.7536) (-100.1584, -31.1753) knots 0 0 0 1 2 2 2
  line L53 (-100.1584, -31.1753) -> (-94.5464, -31.1753)
  line L54 (-94.5464, -31.1753) -> (-94.5464, -32.4405)
  line L55 (-94.5464, -32.4405) -> (-102.0561, -32.4405)
  line L56 (-102.0561, -32.4405) -> (-102.0561, -31.1753)
  line L57 (-102.0561, -31.1753) -> (-101.2289, -31.1753)
  spline S79 degree 2 poles (-101.2289, -31.1753) (-101.7236, -30.6806) (-102.267, -29.7074) (-102.267, -29.1235) knots 0 0 0 1 2 2 2
  spline S80 degree 2 poles (-102.267, -29.1235) (-102.267, -28.4585) (-101.6587, -27.4285) (-100.9694, -27.1609) knots 0 0 0 1 2 2 2
  spline S81 degree 2 poles (-100.9694, -27.1609) (-101.6101, -26.5851) (-102.267, -25.4984) (-102.267, -24.8658) knots 0 0 0 1 2 2 2
  spline S82 degree 2 poles (-102.267, -24.8658) (-102.267, -24.3792) (-101.9669, -23.5845) (-101.6263, -23.2925) knots 0 0 0 1 2 2 2
  spline S83 degree 2 poles (-101.6263, -23.2925) (-101.2857, -22.9924) (-100.2638, -22.6599) (-99.4934, -22.6599) knots 0 0 0 1 2 2 2
  line L58 (-99.4934, -22.6599) -> (-94.5464, -22.6599)
  line L59 (-94.5464, -22.6599) -> (-94.5464, -23.9251)
  point P0 (0, 0)
  dimension "d115" = 5
  dimension "d116" = 75
  dimension "d117" = 10
  constraints: 2 other
  measures "d115" distance between parallel lines of L4 L0
  measures "d116" distance between parallel lines of L3 L1
  measures "d117" distance between parallel lines of L5 L3
extrude "Extrusion14" cut sketch "Sketch14" against normal blind 1.5
body "Solid1"
